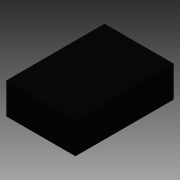
# Autodesk Inventor part: BQ24210DQCT
Saved by Autodesk Inventor 2015 SP1 (Build 190203100, 203)
## iProperties
Created: 2015-10-19
Part Number: BQ24210DQCT
Material: Generic
Document SubType Name: Modeling
Designer: Kartikye
Density: 1 g/cm^3
Appearance: SON50P200X300X80-11N, BQ24210DQCT
Author: Kartikye
Autodesk Inventor part; units mm, degrees
ref_plane "YZ Plane" through (0, 0, 0) normal (1, 0, 0) x (0, 1, 0)
ref_plane "XZ Plane" through (0, 0, 0) normal (0, 1, 0) x (-1, 0, 0)
ref_plane "XY Plane" through (0, 0, 0) normal (0, 0, 1) x (1, 0, 0)
sketch "SON50P200X300X80-11N, BQ24210DQCT_114" plane through (0, 0, 0) normal (0, 0, 1) x (1, 0, 0)
  line L0 (-1.1176, 1.5494) -> (1.1176, 1.5494)
  line L1 (1.1176, 1.5494) -> (1.1176, -1.6256)
  line L2 (1.1176, -1.6256) -> (-1.1176, -1.6256)
  line L3 (-1.1176, -1.6256) -> (-1.1176, 1.5494)
  constraints: 8 end point
extrude "Extrusion1" add sketch "SON50P200X300X80-11N, BQ24210DQCT_114" along normal blind 1
body "Solid1"
